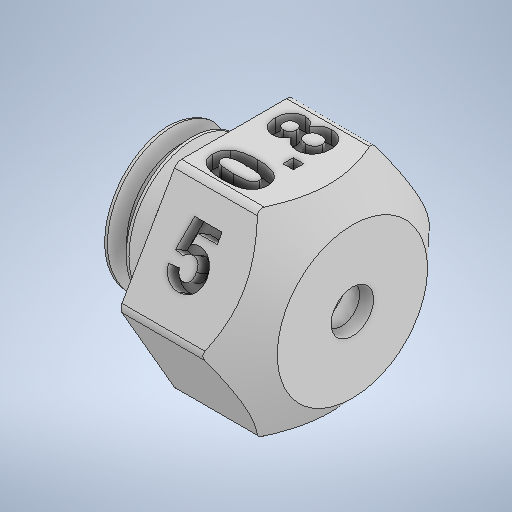
# Autodesk Inventor part: Part1
Saved by Autodesk Inventor 2025.2 (Build 292293000, 293)
## iProperties
Created: 2026-03-09
Part Number: Part1
Material: Generic
Document SubType Name: Modeling
Designer: Simon
Density: 1 g/cm^3
Appearance: Default
Author: Simon
Autodesk Inventor part; units mm, degrees
ref_plane "YZ Plane" through (0, 0, 0) normal (1, 0, 0) x (0, 1, 0)
ref_plane "XZ Plane" through (0, 0, 0) normal (0, 1, 0) x (-1, 0, 0)
ref_plane "XY Plane" through (0, 0, 0) normal (0, 0, 1) x (1, 0, 0)
sketch "Sketch1" plane through (0, 0, 0) normal (0, 0, 1) x (1, 0, 0)
  line L0 (0, 0) -> (0, 1.25)
  line L1 (0, 1.25) -> (50, 1.25)
  line L2 (0, 0) -> (0, 0.6806)
  line L3 (0, 0.6806) -> (50, 0.6806)
  line L4 (0, 0) -> (0, 0.7902)
  line L5 (0, 0.7902) -> (50, 0.7902)
  line L6 (0, 0) -> (0, 2.5)
  line L7 (0, 2.5) -> (2.5, 2.5)
  line L8 (2.5, 2.5) -> (2.5, 1.25)
  line L9 (2.5, 1.25) -> (2.5, 4.25)
  line L10 (2.5, 1.25) -> (6.7109, 1.25) construction
  line L11 (2.5, 4.25) -> (5.5, 4.25)
  line L12 (5.5, 4.25) -> (5.5, 1.25)
  line L13 (5.5, 1.25) -> (6.4863, 0.6806)
  line L14 (5.5, 1.25) -> (9.25, 1.25) construction
  line L15 (6.4863, 0.6806) -> (6.8955, 0.7902)
  line L16 (6.4863, 0.6806) -> (6.91, 0.6806) construction
  line L17 (6.8955, 0.7902) -> (6.8955, 2.7902)
  line L18 (6.8955, 2.7902) -> (5.5, 4.25)
  line L19 (0, 0) -> (50, 0)
  dimension "d0" = 1.25
  dimension "d1" = 50
  dimension "d2" = 0.6806
  dimension "d3" = 0.7902
  dimension "d4" = 2.5
  dimension "d5" = 2.5
  dimension "d6" = 3
  dimension "d8" = 3
  dimension "d9" = 30
  dimension "d10" = 15
  dimension "d12" = 2
  dimension "d13" = 50
  constraints: 40 end point, 7 perpendicular, 7 point on line, 5 horizontal, 2 vertical, 1 equal length
  measures "d0" distance of L0.start L0.end
  measures "d1" distance of L0.end L1.end
  measures "d2" distance of L0.start L2.end
  measures "d3" distance of L0.start L4.end
  measures "d4" distance of L0.start L6.end
  measures "d5" distance of L6.end L7.end
  measures "d6" distance of L8.end L9.end
  measures "d8" distance of L9.end L11.end
  measures "d9" angle of L13 L14
  measures "d10" angle of L16 L15
  measures "d12" distance of L15.end L17.end
  measures "d13" distance of L0.start L19.end
revolve "Revolution1" add sketch "Sketch1" angle 360 about axis through (0, 0, 0) along (1, 0, 0) contours L13 L5 L15 | L6 L7 L8 L1 | L13 L1 L17 L5 | L8 L9 L11 L12 L1 | L12 L18 L17 L1
sketch "Sketch2" plane through (2.5, 0, 0) normal (-1, 0, 0) x (0, 0, 1)
  circle A0 centre (0, 0) radius 4.25 projected
  line L0 (-4.25, 0) -> (4.25, 0)
  circle A1 centre (0, 0) radius 0.6806 projected
  line L1 (4.25, 0) -> (2.125, -3.6806)
  line L2 (2.125, -3.6806) -> (-2.125, -3.6806)
  line L3 (-2.125, -3.6806) -> (-4.25, 0)
  line L4 (-4.25, 0) -> (-2.125, 3.6806)
  line L5 (-2.125, 3.6806) -> (2.125, 3.6806)
  line L6 (2.125, 3.6806) -> (4.25, 0)
  circle A2 centre (0, 0) radius 1.25
  constraints: 14 end point, 2 coincident, 2 point on circle, 1 centre point, 1 horizontal, 13 other
extrude "Extrusion1" cut sketch "Sketch2" against normal through all contours L6 A0 | A0 L1 | L5 A0 | A0 L2 | L4 A0 | A0 L3
fillet "Fillet1" radius 0.3 6 edges at (4, 3.6806, 2.125) (4, 3.6806, -2.125) (4, 0, -4.25) (4, -3.6806, -2.125) (4, -3.6806, 2.125) (4, 0, 4.25)
sketch "Sketch3" plane through (0, 0, 0) normal (0, 0, 1) x (1, 0, 0)
  line L0 (-0.35, 1.8938) -> (0.45, 1.8938)
  line L1 (-0.35, 1.8938) -> (0.05, 2.5866)
  line L2 (-0.35, 1.8938) -> (0.45, 1.8938) construction
  line L3 (0.05, 2.5866) -> (0.45, 1.8938)
  line L4 (-0.0972, 3.8266) -> (0.7028, 3.8266) construction
  line L5 (0.05, 2.5866) -> (0.05, 1.8938)
  line L6 (0.05, 1.8938) -> (0.05, 2.0671)
  line L7 (0.05, 2.0671) -> (0.45, 2.0671)
  line L8 (0.45, 2.0671) -> (-0.35, 2.0671)
  line L9 (0.05, 2.5866) -> (0.05, 2.5)
  line L10 (0.05, 2.5) -> (0.45, 2.5)
  line L11 (0.45, 2.5) -> (-0.35, 2.5)
  line L12 (-0.35, 1.8938) -> (-1.15, 1.8938)
  line L13 (0.05, 2.5866) -> (-0.75, 2.5866)
  line L14 (-0.75, 2.5866) -> (-1.15, 1.8938)
  line L15 (-0.35, 1.8938) -> (-0.75, 2.5866)
  line L16 (-0.35, 2.0671) -> (-1.15, 2.0671)
  line L17 (-0.35, 2.5) -> (-0.8, 2.5)
  line L18 (-0.75, 2.5866) -> (-0.75, 1.8938)
  line L19 (-0.35, 1.8938) -> (-0.35, 1.9938)
  circle A0 centre (-0.35, 2.0938) radius 0.1
  line L20 (-0.4077, 1.9938) -> (-0.2923, 1.9938)
  line L21 (0, 2.5) -> (2.5, 2.5) projected
  line L22 (0, 2.5) -> (-0.7, 2.5)
  line L23 (-0.7, 2.5) -> (-0.4366, 2.0438)
  line L24 (-0.4366, 2.0438) -> (-0.2634, 2.0438)
  line L25 (-0.2634, 2.0438) -> (0, 2.5)
  circle A1 centre (-0.35, 2.0938) radius 0.1
  point P0 (0, 0)
  point P1 (0, 2.5)
  dimension "d18" = 0.8
  dimension "d19" = 60
  dimension "d20" = 60
  dimension "d21" = 0.1732
  dimension "d22" = 0.0866
  dimension "d23" = 0.8
  dimension "d24" = 0.1
  dimension "d25" = 0.8
  constraints: 50 end point, 13 point on line, 7 horizontal, 4 tangent, 3 midpoint, 2 centre point, 2 equal length, 2 perpendicular, 2 point on circle, 1 coincident, 1 collinear, 1 concentric, 1 parallel, 1 vertical
  measures "d18" distance of L2.start L0.end
  measures "d19" angle of L2 L1
  measures "d20" angle of L3 L4
  measures "d21" distance of L6.start L7.start
  measures "d22" distance of L3.start L10.start
  measures "d23" distance of L2.start L12.end
  measures "d24" distance of L2.start L19.end
  measures "d25" distance between parallel lines of L5 L18
coil "Coil1" sketch "Sketch3" operation cut axis through (-10, 0, 0) along (1, 0, 0) pitch 0.8 turns 4 hand right contours A0 L24 | L24 L15 L16 L8 L1 | A0 L15 L17 L11 L1 | L8 L16 A0
extrude "Extrusion2" add sketch "Sketch2" against normal blind 3 contours L1 L2 L3 L0 A2 | L0 A2 L4 L5 L6
fillet "Fillet2" radius 0.3 6 edges at (4, 3.6806, -2.125) (4, 3.6806, 2.125) (4, 0, 4.25) (4, -3.6806, 2.125) (4, -3.6806, -2.125) (4, 0, -4.25)
sketch "Sketch4" plane through (2.5, 3.6806, 1.9518) normal (0, 1, 0) x (1, 0, 0)
  line L0 (0.4064, -0.0137) -> (0.4064, 4.3493) construction
  line L1 (0.4064, 4.3493) -> (2.509, 4.3493) construction
  line L2 (2.509, 4.3493) -> (2.509, -0.0137) construction
  line L3 (2.509, -0.0137) -> (0.4064, -0.0137) construction
  spline S0 degree 2 poles (0.4064, 0.753) (0.4064, 1.0442) (0.6137, 1.2073) knots 0 0 0 1 1 1
  spline S1 degree 2 poles (0.6137, 1.2073) (0.8592, 1.4024) (1.4277, 1.4024) knots 0 0 0 1 1 1
  spline S2 degree 2 poles (1.4277, 1.4024) (1.9948, 1.4024) (2.2433, 1.2058) knots 0 0 0 1 1 1
  spline S3 degree 2 poles (2.2433, 1.2058) (2.4476, 1.0442) (2.4476, 0.753) knots 0 0 0 1 1 1
  spline S4 degree 2 poles (2.4476, 0.753) (2.4476, 0.4604) (1.9994, 0.1036) (1.4232, 0.1036) knots 0 0 0 1 2 2 2
  spline S5 degree 2 poles (1.4232, 0.1036) (0.8592, 0.1036) (0.6107, 0.3003) knots 0 0 0 1 1 1
  spline S6 degree 2 poles (0.6107, 0.3003) (0.4064, 0.4619) (0.4064, 0.753) knots 0 0 0 1 1 1
  spline S7 degree 2 poles (0.725, 0.753) (0.725, 0.6829) (0.8134, 0.5747) (0.9277, 0.5442) knots 0 0 0 1 2 2 2
  spline S8 degree 2 poles (0.9277, 0.5442) (1.0756, 0.5046) (1.4277, 0.5046) knots 0 0 0 1 1 1
  spline S9 degree 2 poles (1.4277, 0.5046) (1.7784, 0.5046) (2.0421, 0.5762) (2.129, 0.6829) (2.129, 0.753) knots 0 0 0 1 2 3 3 3
  spline S10 degree 2 poles (2.129, 0.753) (2.129, 0.8232) (2.0406, 0.9314) (1.9262, 0.9619) knots 0 0 0 1 2 2 2
  spline S11 degree 2 poles (1.9262, 0.9619) (1.7784, 1.0015) (1.4277, 1.0015) knots 0 0 0 1 1 1
  spline S12 degree 2 poles (1.4277, 1.0015) (1.0756, 1.0015) (0.8134, 0.9299) (0.725, 0.8232) (0.725, 0.753) knots 0 0 0 1 2 3 3 3
  line L4 (2.414, 1.7393) -> (2.0299, 1.7393)
  line L5 (2.0299, 1.7393) -> (2.0299, 2.1235)
  line L6 (2.0299, 2.1235) -> (2.414, 2.1235)
  line L7 (2.414, 2.1235) -> (2.414, 1.7393)
  spline S13 degree 2 poles (1.3348, 2.7622) (1.2723, 2.6143) (1.0527, 2.4786) (0.9217, 2.4786) knots 0 0 0 1 2 2 2
  spline S14 degree 2 poles (0.9217, 2.4786) (0.6976, 2.4786) (0.4064, 2.7911) (0.4064, 3.0793) knots 0 0 0 1 2 2 2
  spline S15 degree 2 poles (0.4064, 3.0793) (0.4064, 3.3643) (0.6976, 3.6799) (0.9217, 3.6799) knots 0 0 0 1 2 2 2
  spline S16 degree 2 poles (0.9217, 3.6799) (1.0604, 3.6799) (1.2768, 3.535) (1.3348, 3.4039) knots 0 0 0 1 2 2 2
  spline S17 degree 2 poles (1.3348, 3.4039) (1.4018, 3.5701) (1.6579, 3.7439) (1.8256, 3.7439) knots 0 0 0 1 2 2 2
  spline S18 degree 2 poles (1.8256, 3.7439) (2.1031, 3.7439) (2.4491, 3.3902) (2.4491, 3.0975) knots 0 0 0 1 2 2 2
  spline S19 degree 2 poles (2.4491, 3.0975) (2.4491, 2.8247) (2.3058, 2.6433) knots 0 0 0 1 1 1
  spline S20 degree 2 poles (2.3058, 2.6433) (2.1366, 2.4283) (1.8424, 2.4283) knots 0 0 0 1 1 1
  spline S21 degree 2 poles (1.8424, 2.4283) (1.6793, 2.4283) (1.4079, 2.5899) (1.3348, 2.7622) knots 0 0 0 1 2 2 2
  spline S22 degree 2 poles (1.8058, 2.8064) (1.9643, 2.8064) (2.1412, 2.968) (2.1412, 3.0899) knots 0 0 0 1 2 2 2
  spline S23 degree 2 poles (2.1412, 3.0899) (2.1412, 3.2088) (1.9704, 3.3643) (1.8088, 3.3643) knots 0 0 0 1 2 2 2
  spline S24 degree 2 poles (1.8088, 3.3643) (1.6686, 3.3643) (1.4979, 3.2058) (1.4979, 3.0854) knots 0 0 0 1 2 2 2
  spline S25 degree 2 poles (1.4979, 3.0854) (1.4979, 2.9436) (1.6915, 2.8064) (1.8058, 2.8064) knots 0 0 0 1 2 2 2
  spline S26 degree 2 poles (0.9491, 2.8414) (1.0634, 2.8414) (1.1915, 2.971) (1.1915, 3.0793) knots 0 0 0 1 2 2 2
  spline S27 degree 2 poles (1.1915, 3.0793) (1.1915, 3.189) (1.0619, 3.3201) (0.9476, 3.3201) knots 0 0 0 1 2 2 2
  spline S28 degree 2 poles (0.9476, 3.3201) (0.8409, 3.3201) (0.7113, 3.1905) (0.7113, 3.0838) knots 0 0 0 1 2 2 2
  spline S29 degree 2 poles (0.7113, 3.0838) (0.7113, 2.9725) (0.8424, 2.8414) (0.9491, 2.8414) knots 0 0 0 1 2 2 2
  point P0 (-2.5, 1.9518)
  constraints: 2 other
extrude "Extrusion3" cut sketch "Sketch4" against normal blind 0.5
sketch "Sketch5" plane through (2.5, 0.15, 4.1634) normal (0, 0.5, 0.866) x (1, 0, 0)
  line L0 (0.8204, 3.039) -> (2.3737, 3.039) construction
  line L1 (2.3737, 3.039) -> (2.3737, 1.0313) construction
  line L2 (2.3737, 1.0313) -> (0.8204, 1.0313) construction
  line L3 (0.8204, 1.0313) -> (0.8204, 3.039) construction
  line L4 (0.8204, 3.039) -> (2.3737, 3.039) construction
  line L5 (2.3737, 3.039) -> (2.3737, 1.0313) construction
  line L6 (2.3737, 1.0313) -> (0.8204, 1.0313) construction
  line L7 (0.8204, 1.0313) -> (0.8204, 3.039) construction
  line L8 (0.9438, 1.5786) -> (1.3265, 1.6182)
  spline S0 degree 2 poles (1.3265, 1.6182) (1.3432, 1.4887) (1.5033, 1.3377) (1.6085, 1.3377) knots 0 0 0 1 2 2 2
  spline S1 degree 2 poles (1.6085, 1.3377) (1.7289, 1.3377) (1.8951, 1.5329) (1.8951, 1.731) knots 0 0 0 1 2 2 2
  spline S2 degree 2 poles (1.8951, 1.731) (1.8951, 1.9155) (1.7289, 2.0999) (1.5963, 2.0999) knots 0 0 0 1 2 2 2
  spline S3 degree 2 poles (1.5963, 2.0999) (1.4316, 2.0999) (1.3005, 1.9536) knots 0 0 0 1 1 1
  line L9 (1.3005, 1.9536) -> (0.9896, 1.9993)
  line L10 (0.9896, 1.9993) -> (1.1862, 3.039)
  line L11 (1.1862, 3.039) -> (2.2015, 3.039)
  line L12 (2.2015, 3.039) -> (2.2015, 2.6807)
  line L13 (2.2015, 2.6807) -> (1.4774, 2.6807)
  line L14 (1.4774, 2.6807) -> (1.4164, 2.3408)
  spline S4 degree 2 poles (1.4164, 2.3408) (1.5444, 2.4048) (1.6786, 2.4048) knots 0 0 0 1 1 1
  spline S5 degree 2 poles (1.6786, 2.4048) (1.9347, 2.4048) (2.2899, 2.0329) (2.2899, 1.7371) knots 0 0 0 1 2 2 2
  spline S6 degree 2 poles (2.2899, 1.7371) (2.2899, 1.4902) (2.1466, 1.2966) knots 0 0 0 1 1 1
  spline S7 degree 2 poles (2.1466, 1.2966) (1.9515, 1.0313) (1.6039, 1.0313) knots 0 0 0 1 1 1
  spline S8 degree 2 poles (1.6039, 1.0313) (1.328, 1.0313) (0.9774, 1.3286) (0.9438, 1.5786) knots 0 0 0 1 2 2 2
  point P0 (-2.5, 1.9518)
  constraints: 4 other
extrude "Extrusion4" cut sketch "Sketch5" against normal blind 0.5
body "Solid1"
